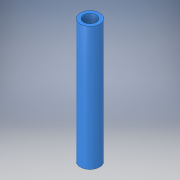
# Autodesk Inventor part: Stewart-Rod-Pipe-Small
Saved by Autodesk Inventor 2018.2 (Build 222227000, 227)
## iProperties
Created: 2018-02-18
Part Number: Stewart-Rod-Pipe-Small
Material: Generisch
Document SubType Name: Modeling
Designer: JochenAlt
Density: 1 g/cm^3
Appearance: Vorgabe
Author: JochenAlt
Autodesk Inventor part; units mm, degrees
ref_plane "YZ Plane" through (0, 0, 0) normal (1, 0, 0) x (0, 1, 0)
ref_plane "XZ Plane" through (0, 0, 0) normal (0, 1, 0) x (-1, 0, 0)
ref_plane "XY Plane" through (0, 0, 0) normal (0, 0, 1) x (1, 0, 0)
sketch "Skizze1" plane through (0, 0, 0) normal (0, 0, 1) x (1, 0, 0)
  circle A0 centre (0, 0) radius 1.55
  circle A1 centre (0, 0) radius 2.35
  dimension "d0" = 0.8
  dimension "d1" = 3.1
  constraints: 2 centre point, 2 coincident
  measures "d0" radial gap between concentric circles of A1 A0
  measures "d1" diameter of A0
extrude "Extrusion1" add sketch "Skizze1" along normal blind 30
